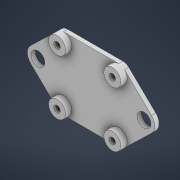
# Autodesk Inventor part: adapter_board_mount
Saved by Autodesk Inventor 2021 (Build 250183000, 183)
## iProperties
Created: 2024-07-10
Part Number: adapter_board_mount
Material: Generic
Document SubType Name: Modeling
Designer: loren
Density: 1 g/cm^3
Appearance: Default
Author: loren
Autodesk Inventor part; units mm, degrees
ref_plane "YZ Plane" through (0, 0, 0) normal (1, 0, 0) x (0, 1, 0)
ref_plane "XZ Plane" through (0, 0, 0) normal (0, 1, 0) x (-1, 0, 0)
ref_plane "XY Plane" through (0, 0, 0) normal (0, 0, 1) x (1, 0, 0)
sketch "Sketch1" plane through (0, 0, 0) normal (0, 0, 1) x (1, 0, 0)
  line L0 (-13, 13) -> (13, 13) construction
  line L1 (13, 13) -> (13, -13) construction
  line L2 (13, -13) -> (-13, -13) construction
  line L3 (-13, -13) -> (-13, 13) construction
  circle A0 centre (-13, 13) radius 1.5
  circle A1 centre (-13, -13) radius 1.5
  circle A2 centre (-13, 13) radius 4
  circle A3 centre (-13, -13) radius 4
  line L4 (-15.7812, 15.8749) -> (-28.4765, 3.5936)
  arc A4 (-28.4765, 3.5936) -> (-28.4765, -3.5936) centre (-25, 0) ccw
  line L5 (-28.4765, -3.5936) -> (-15.7812, -15.8749)
  line L6 (-13, 17) -> (0, 17)
  line L7 (0, 17) -> (0, -17)
  line L8 (0, -17) -> (-13, -17)
  circle A5 centre (-25, 0) radius 3.25
  point P0 (0, 0)
  point P1 (0, 13)
  point P2 (-13, 0)
  point P3 (0, 0)
  dimension "d0" = 26
  dimension "d1" = 3
  dimension "d3" = 8
  dimension "d5" = 10
  dimension "d6" = 25
  dimension "d7" = 6.5
  constraints: 18 end point, 6 centre point, 6 coincident, 6 point on circle, 6 tangent, 4 perpendicular, 3 midpoint, 2 equal radius, 2 horizontal, 2 horizontal alignment, 2 parallel, 1 vertical alignment
  measures "d0" distance of L0.start L0.end
  measures "d1" diameter of A0
  measures "d3" diameter of A2
  measures "d5" diameter of A4
  measures "d6" distance from line of L7 A4.centre
  measures "d7" diameter of A5
extrude "Extrusion1" add sketch "Sketch1" along normal blind 2
extrude "Extrusion2" add sketch "Sketch1" along normal blind 5 contours A2 | A3
mirror "Mirror1" about plane through (0, 0, 0) normal (1, 0, 0)
body "Solid1"
